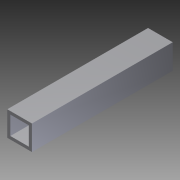
# Autodesk Inventor part: internalframeconnector
Saved by Autodesk Inventor 2012 (Build 160160000, 160)
## iProperties
Created: 2012-01-12
Part Number: internalframeconnector
Material: Default
Document SubType Name: Modeling
Designer: William
Density: 1 g/cm^3
Author: William
Autodesk Inventor part; units mm, degrees
ref_plane "YZ Plane" through (0, 0, 0) normal (1, 0, 0) x (0, 1, 0)
ref_plane "XZ Plane" through (0, 0, 0) normal (0, 1, 0) x (-1, 0, 0)
ref_plane "XY Plane" through (0, 0, 0) normal (0, 0, 1) x (1, 0, 0)
sketch "Sketch1" plane through (0, 0, 0) normal (0, 0, 1) x (1, 0, 0)
  line L0 (-14.0233, 19.5756) -> (11.3767, 19.5756)
  line L1 (11.3767, 19.5756) -> (11.3767, -5.8244)
  line L2 (11.3767, -5.8244) -> (-14.0233, -5.8244)
  line L3 (-14.0233, -5.8244) -> (-14.0233, 19.5756)
  line L4 (-10.8483, 16.4006) -> (8.2017, 16.4006)
  line L5 (8.2017, 16.4006) -> (8.2017, -2.6494)
  line L6 (8.2017, -2.6494) -> (-10.8483, -2.6494)
  line L7 (-10.8483, -2.6494) -> (-10.8483, 16.4006)
  point P0 (0, 0)
  dimension "d0" = 3.175
  dimension "d1" = 3.175
  dimension "d2" = 3.175
  dimension "d3" = 3.175
  dimension "d4" = 25.4
  dimension "d5" = 25.4
  constraints: 16 end point, 4 parallel, 2 horizontal, 2 perpendicular
  measures "d0" distance between parallel lines of L0 L4
  measures "d1" distance between parallel lines of L1 L5
  measures "d2" distance between parallel lines of L3 L7
  measures "d3" distance between parallel lines of L2 L6
  measures "d4" distance of L0.start L0.end
  measures "d5" distance of L2.end L0.start
extrude "Extrusion1" add sketch "Sketch1" along normal blind 144.8308
equation "\"d1\" = d3"
equation "\"d2\" = d0"
equation "\"d3\" = d2"
equation "\"d5\" = d4"
body "Solid1"
